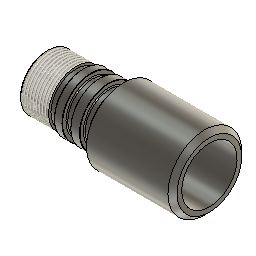
penetrator_sensor_Atlas_K1_0 (Autodesk Fusion 360 design; units mm, degrees)
Autodesk Fusion 360 part; units mm, degrees
sketch "Sketch1" plane through (0, 0, 0) normal (0, 1, 0) x (1, 0, 0)
  line L0 (50, -5.9975) -> (50, -0.0016) construction
  line L1 (0, -6.5) -> (0, -9)
  line L2 (0, -9) -> (38.6, -9)
  line L3 (43.6, -8) -> (46.3, -8)
  line L4 (46.3, -8) -> (46.3, -9.5)
  line L5 (46.3, -9.5) -> (49.3, -9.5)
  line L6 (49.3, -9.5) -> (49.3, -8)
  line L7 (49.3, -8) -> (52, -8)
  line L8 (52, -8) -> (52, -9.5)
  line L9 (52, -9.5) -> (54, -9.5)
  line L10 (54, -9.5) -> (54, -12)
  line L11 (54, -12) -> (82, -12)
  line L12 (82, -12) -> (82, -9)
  line L13 (82, -9) -> (59, -9)
  line L14 (59, -9) -> (59, -6.5)
  line L15 (59, -6.5) -> (0, -6.5)
  line L16 (40.6, -9) -> (40.6, -9.5)
  line L17 (40.6, -9.5) -> (43.6, -9.5)
  line L18 (43.6, -9.5) -> (43.6, -8)
  line L19 (40.6, -9) -> (40.6, -8.2)
  line L20 (40.6, -8.2) -> (38.6, -8.2)
  line L21 (38.6, -8.2) -> (38.6, -9)
  line L22 (102.7, 1.5) -> (99.7, 1.5) construction
  line L23 (99.7, -1.5) -> (102.7, -1.5) construction
  line L24 (98.2, 0) -> (104.2, 0) construction
  arc A0 (102.7, -1.5) -> (102.7, 1.5) centre (102.7, 0) ccw construction
  arc A1 (99.7, 1.5) -> (99.7, -1.5) centre (99.7, 0) ccw construction
  line L25 (0, 0) -> (12.5649, 0) construction
  line L26 (110, -6) -> (110, 0) construction
  line L27 (0, -6) -> (110, -6) construction
  line L28 (-35.6, -8.1) -> (0, -8.1) construction
  line L29 (0, -8.1) -> (0, -6) construction
  line L30 (-35.6, -8.1) -> (-35.6, -2.5) construction
  line L31 (-35.6, -2.5) -> (-61.6, -1) construction
  line L32 (-61.6, -1) -> (-61.6, 0) construction
  line L33 (54, -12) -> (35, -12) construction
  line L34 (29, -9) -> (29, -8)
  line L35 (0, -8) -> (29, -8)
  line L36 (29, -8) -> (29, -6.5)
  dimension "d6" = 54
  dimension "d7" = 5
  dimension "d9" = 6.5
  dimension "d10" = 9
  dimension "d11" = 12
  dimension "d13" = 2.7
  dimension "d14" = 3
  dimension "d15" = 2
  dimension "d26" = 9
  dimension "d29" = 9.5
  dimension "d30" = 3
  dimension "d31" = 1.5
  dimension "d34" = 13.4
  dimension "d35" = 8.2
  dimension "d36" = 2
  dimension "d48" = 3
  dimension "d49" = 6
  dimension "d51" = 6
  dimension "d52" = 8.1
  dimension "d53" = 110
  dimension "d54" = 35.6
  dimension "d55" = 26
  dimension "d56" = 2.5
  dimension "d57" = 1
  dimension "d58" = 19
  dimension "d60" = 96.6
  dimension "d61" = 28
  dimension "d62" = 70.6
  dimension "d63" = 8
  dimension "d64" = 6
  dimension "d65" = 16.2
  dimension "d67" = 28
  dimension "d68" = 29
  constraint perpendicular L3 L4
  constraint perpendicular L4 L5
  constraint perpendicular L3 L6
  constraint perpendicular L6 L7
  constraint perpendicular L7 L8
  constraint perpendicular L8 L9
  constraint perpendicular L9 L10
  constraint perpendicular L0 L11
  constraint perpendicular L11 L12
  constraint perpendicular L0 L13
  constraint perpendicular L11 L14
  constraint horizontal L15
  constraint equal L3 L7
  constraint collinear L5 L9
  constraint perpendicular L2 L16
  constraint perpendicular L16 L17
  constraint collinear L5 L17
  constraint vertical L18
  constraint collinear L3 L7
  constraint perpendicular L2 L19
  constraint perpendicular L19 L20
  constraint perpendicular L2 L21
  constraint tangent L23 A0
  constraint tangent L22 A0
  constraint parallel L22 L23
  constraint tangent L22 A1
  constraint tangent L23 A1
  constraint midpoint L24.start A1
  constraint midpoint L24.end A0
  constraint coincident L25.start origin
  constraint horizontal L27
  constraint perpendicular L28 L30
  constraint perpendicular L28 L32
  constraint horizontal L25.start L32.end
  constraint vertical L29
  constraint vertical L25.start L27.start
  constraint horizontal L33
  constraint vertical L25.start L1.end
  constraint horizontal L2
  constraint coincident L2 L34.start
  constraint perpendicular L2 L34
  constraint coincident L1 L35.start
  constraint horizontal L35
  constraint vertical L1
  constraint vertical L26
  constraint coincident L15 L36.end
  constraint perpendicular L15 L36
  measures "d6" distance of L1.end L10
  measures "d7" distance of L10 L14
  measures "d9" distance of L25.start L15
  measures "d10" distance of L25.start L13
  measures "d11" distance of L25.start L11
  measures "d13" distance of L3.start L3.end
  measures "d14" distance of L4.end L5.end
  measures "d15" distance of L8.end L9.end
  measures "d26" distance of L25.start L2
  measures "d29" distance of L25.start L5
  measures "d30" distance of L16.end L17.end
  measures "d31" distance of L3.start L17.end
  measures "d34" distance of L10 L16
  measures "d35" distance of L25.start L20
  measures "d36" distance of L19.end L20.end
  measures "d48" distance of L22 L23
  measures "d49" distance of L24.start L24.end
  measures "d51" distance of L25 L27
  measures "d52" distance of L25 L28
  measures "d53" distance of L25.start L26
  measures "d54" distance of L28.start L28.end
  measures "d55" horizontal distance of L30.end L31.end
  measures "d56" vertical distance of L25.start L30.end
  measures "d57" distance of L31.end L32.end
  measures "d58" distance of L10.end L33.end
  measures "d60" horizontal distance of L31.end L33.end
  measures "d61" distance of L10.end L11.end
  measures "d62" horizontal distance of L28.start L33.end
  measures "d63" distance of L25.start L35
  measures "d64" distance of L33.end L34
  measures "d65" distance of L12 L24.start
  measures "d67" horizontal distance of L11.end L26.end
  measures "d68" distance of L1.end L34.start
revolve "Revolve1" add sketch "Sketch1" angle 360 about axis through (1.75, 0, 0) along (1, 0, 0) contours L2 L3 L4 L5 L6 L7 L8 L9 L10 L11 L12 L13 L14 L15 L16 L17 L18 L19 L20 L21 L34 L36
fillet "Fillet2" radius 0.3 2 faces at (44.5, 0.3988, 7.9901) (50.2, 0.3988, 7.9901)
chamfer "Chamfer2" distance 1.5 angle 45 1 edges at (82, -4.3394, -11.1879)
thread "Thread1" "ISO Metric profile 18.0 M18x1 6g" major diameter 17.884 minor diameter 16.741 pitch 1 angle 60 resizes the face on face at (32.2, 0.8961, 8.9553)
chamfer "Chamfer3" distance 0.5 angle 45 1 edges at (29, -3.2336, -8.3369)
fillet "Fillet3" radius 1 1 edges at (59, -3.2545, -8.3909)
chamfer "Chamfer4" distance 0.5 angle 45 1 edges at (40.6, -3.4353, -8.8571)
fillet "Fillet4" radius 0.1 2 edges at (43.6, -3.4353, -8.8571) (52, -3.4353, -8.8571) 1 faces at (47.3, 0.4735, 9.4882)
equation "d6 = 29 mm + 25 mm"
equation "d61 = 21.00 mm + 7 mm"
equation "d63 = ( 16 / 2 ) * 1 mm"
